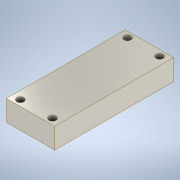
# Autodesk Inventor part: openCM904
Saved by Autodesk Inventor 2021 (Build 250183000, 183)
## iProperties
Created: 2020-11-13
Part Number: openCM904
Material: Titanium
Document SubType Name: Modeling
Designer: Paco
Density: 0.642143 g/cm^3
Appearance: Titanium
Mass: 13 g
Surface Area: 62.4275 cm^2
Volume: 20.2447 cm^3
Author: Paco
Autodesk Inventor part; units mm, degrees
ref_plane "YZ Plane" through (0, 0, 0) normal (1, 0, 0) x (0, 1, 0)
ref_plane "XZ Plane" through (0, 0, 0) normal (0, 1, 0) x (-1, 0, 0)
ref_plane "XY Plane" through (0, 0, 0) normal (0, 0, 1) x (1, 0, 0)
sketch "Sketch1" plane through (0, 0, 0) normal (0, 1, 0) x (-1, 0, 0)
  line L0 (45.232, 28.7572) -> (18.232, 28.7572)
  line L1 (18.232, 28.7572) -> (18.232, -37.7428)
  line L2 (18.232, -37.7428) -> (45.232, -37.7428)
  line L3 (45.232, -37.7428) -> (45.232, 28.7572)
  circle A0 centre (40.732, -34.4928) radius 2
  circle A1 centre (22.732, -34.4928) radius 2
  circle A2 centre (40.732, 25.5072) radius 2
  circle A3 centre (22.732, 25.5072) radius 2
  point P0 (0, 0)
  dimension "d0" = 66.5
  dimension "d1" = 27
  dimension "d2" = 4
  dimension "d3" = 4
  dimension "d4" = 18
  dimension "d5" = 4.5
  dimension "d6" = 4
  dimension "d7" = 60
  dimension "d9" = 4
  dimension "d10" = 18
  dimension "d11" = 60
  dimension "d15" = 3.25
  dimension "d16" = 3.25
  constraints: 8 end point, 4 centre point, 2 parallel, 1 horizontal, 1 perpendicular
  measures "d0" distance of L2.end L0.start
  measures "d1" distance of L1.end L2.end
  measures "d2" diameter of A0
  measures "d3" diameter of A1
  measures "d4" distance of A1.centre A0.centre
  measures "d5" distance from line of L3 A0.centre
  measures "d6" diameter of A2
  measures "d7" distance of A2.centre A0.centre
  measures "d9" diameter of A3
  measures "d10" distance of A3.centre A2.centre
  measures "d11" distance of A3.centre A1.centre
  measures "d15" distance from line of L2 A0.centre
  measures "d16" distance from line of L0 A2.centre
extrude "Extrusion1" add sketch "Sketch1" along normal blind 11.6
body "Solid1"
